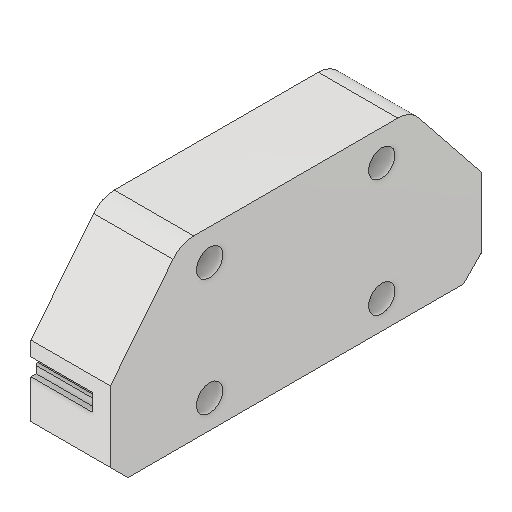
# Autodesk Inventor part: 3DP_PLA_Y_axis_belt_mount
Saved by Autodesk Inventor 2026.1 (Build 301233000, 233)
## iProperties
Created: 2018-07-07
Part Number: 3DP_PLA_Y_axis_belt_mount
Material: ABS Plastic
Document SubType Name: Modeling
Designer: Andrzej
Density: 1.06 g/cm^3
Appearance: Smooth - White
Author: Andrzej
Autodesk Inventor part; units mm, degrees
ref_plane "YZ Plane" through (0, 0, 0) normal (1, 0, 0) x (0, 1, 0)
ref_plane "XZ Plane" through (0, 0, 0) normal (0, 1, 0) x (-1, 0, 0)
ref_plane "XY Plane" through (0, 0, 0) normal (0, 0, 1) x (1, 0, 0)
sketch "Sketch1" plane through (0, 0, 0) normal (1, 0, 0) x (0, 1, 0)
  line L0 (8.9986, 8.0679) -> (-11.0014, 8.0679)
  line L1 (-11.0014, 8.0679) -> (-11.0014, -33.9321)
  line L2 (-11.0014, -33.9321) -> (8.9986, -33.9321)
  line L3 (8.9986, -33.9321) -> (8.9986, 8.0679)
  line L4 (-2.6514, 8.0679) -> (-2.6514, -33.9321)
  line L5 (-4.6014, 8.0679) -> (-4.6014, -33.9321)
  point P0 (0, 0)
  point P1 (5.4986, -3.1821)
  point P2 (-7.8014, -3.1821)
  point P3 (5.4986, -22.6821)
  point P4 (-7.8014, -22.6821)
  dimension "d1" = 42
  dimension "d2" = 1.95
  dimension "d3" = 11.65
  dimension "d4" = 6.4
  dimension "d18" = 11.25
  dimension "d19" = 11.25
  dimension "d20" = 3.5
  dimension "d21" = 3.2
  dimension "d39" = 20
  constraints: 12 end point, 4 point on line, 3 perpendicular, 2 horizontal alignment, 2 parallel, 2 vertical alignment, 1 horizontal
  measures "d1" distance of L1.end L0.end
  measures "d2" distance between parallel lines of L5 L4
  measures "d3" distance between parallel lines of L3 L4
  measures "d4" distance between parallel lines of L1 L5
  measures "d18" distance from line of L0 point (5.499, -3.182)
  measures "d19" distance from line of L2 point (5.499, -22.682)
  measures "d20" distance from line of L3 point (5.499, -3.182)
  measures "d21" distance from line of L1 point (-7.801, -3.182)
  measures "d39" distance between parallel lines of L1 L3
extrude "Extrusion1" add sketch "Sketch1" along normal blind 7 contours L3 L2 L4 L0 | L5 L2 L1 L0
sketch "Sketch2" plane through (7, 0, 0) normal (1, 0, 0) x (0, 0, -1)
  line L0 (-8.0679, 8.9986) -> (-8.0679, -2.6514) projected
  line L1 (-8.0679, -2.6514) -> (33.9321, -2.6514) projected
  line L2 (33.9321, -2.6514) -> (33.9321, 8.9986) projected
  line L3 (33.9321, 8.9986) -> (-8.0679, 8.9986) projected
  line L4 (33.9321, -11.0014) -> (33.9321, -4.6014) projected
  line L5 (33.9321, -4.6014) -> (-8.0679, -4.6014) projected
  line L6 (-8.0679, -4.6014) -> (-8.0679, -11.0014) projected
  line L7 (-8.0679, -11.0014) -> (33.9321, -11.0014) projected
  line L8 (-8.0679, -2.6514) -> (-8.0679, -4.6014)
  line L9 (33.9321, -2.6514) -> (33.9321, 8.9986) projected
  line L10 (33.9321, -11.0014) -> (33.9321, -4.6014) projected
  line L11 (33.9321, -2.6514) -> (33.9321, -4.6014)
  point P0 (0, 0)
  constraints: 4 end point, 2 vertical
extrude "Extrusion2" add sketch "Sketch2" along normal blind 2
sketch "Sketch3" plane through (0, 0, 0) normal (-1, 0, 0) x (0, 0, 1)
  line L0 (-33.9321, -11.0014) -> (-33.9321, -4.6014) projected
  line L1 (8.0679, -11.0014) -> (-33.9321, -11.0014) projected
  line L2 (8.0679, -4.6014) -> (8.0679, -11.0014) projected
  line L3 (-33.9321, -4.6014) -> (8.0679, -4.6014) projected
  line L4 (8.0679, 8.9986) -> (8.0679, -2.6514) projected
  line L5 (-33.9321, 8.9986) -> (8.0679, 8.9986) projected
  line L6 (-33.9321, -2.6514) -> (-33.9321, 8.9986) projected
  line L7 (8.0679, -2.6514) -> (-33.9321, -2.6514) projected
  line L8 (-33.3321, -4.6014) -> (-32.5321, -4.6014)
  line L9 (-32.5321, -4.6014) -> (-32.5321, -3.6014)
  line L10 (-32.5321, -3.6014) -> (-33.3321, -3.6014)
  line L11 (-33.3321, -3.6014) -> (-33.3321, -4.6014)
  point P0 (0, 0)
  dimension "d9" = 1
  dimension "d10" = 0.8
  dimension "d11" = 0.6
  constraints: 8 end point, 2 parallel, 1 horizontal, 1 perpendicular, 1 point on line
  measures "d9" distance between parallel lines of L3 L10
  measures "d10" distance between parallel lines of L11 L9
  measures "d11" distance between parallel lines of L0 L11
extrude "Extrusion3" add sketch "Sketch3" against normal up to surface (7 mm away) contours L11 L10 L9 L3
fillet "Fillet1" radius 0.2 2 edges at (3.5, -3.6014, -33.3321) (3.5, -3.6014, -32.5321)
pattern_linear "Rectangular Pattern1" count 21 spacing 2 along (0, 0, 1) of "Extrusion3", "Fillet1"
hole "Hole1" at (0, 5.4986, -3.1821) at (0, -7.8014, -3.1821) at (0, -7.8014, -22.6821) at (0, 5.4986, -22.6821) direction (1, 0, 0) diameter 3 end through all
chamfer "Chamfer1" distance 2 angle 45 2 edges at (4.5, -11.0014, 8.0679) (4.5, -11.0014, -33.9321)
chamfer "Chamfer2" distance 10 distance2 8 1 edges at (4.5, 8.9986, -33.9321) measured on face at (5.3333, 5.1153, -33.9321)
chamfer "Chamfer3" distance 10 distance2 8 1 edges at (4.5, 8.9986, 8.0679) measured on face at (5.3333, 5.1153, 8.0679)
fillet "Fillet2" radius 3 2 edges at (4.5, 8.9986, -25.9321) (4.5, 8.9986, 0.0679)
equation "\"d19\" = d18"
equation "\"d21\" = 0.5 * d4"
body "Solid1"
